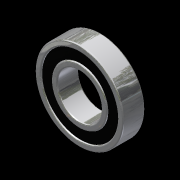
# Autodesk Inventor part: R8-2RS
Saved by Autodesk Inventor 2014 SP1 (Build 180222100, 222)
## iProperties
Created: 2014-04-23
Part Number: R8-2RS
Material: Generic
Document SubType Name: Modeling
Designer: Rauhul Varma
Density: 1 g/cm^3
Appearance: Default
Author: Rauhul Varma
Autodesk Inventor part; units mm, degrees
ref_plane "YZ Plane" through (0, 0, 0) normal (1, 0, 0) x (0, 1, 0)
ref_plane "XZ Plane" through (0, 0, 0) normal (0, 1, 0) x (-1, 0, 0)
ref_plane "XY Plane" through (0, 0, 0) normal (0, 0, 1) x (1, 0, 0)
sketch "Sketch1" plane through (0, 0, 0) normal (0, 0, 1) x (1, 0, 0)
  circle A0 centre (0, 0) radius 6
  circle A1 centre (0, 0) radius 12
  circle A2 centre (0, 0) radius 7.5875
  circle A3 centre (0, 0) radius 10.4125
  dimension "d0" = 12
  dimension "d1" = 24
  dimension "d2" = 15.175
  dimension "d3" = 1.5875
  constraints: 4 centre point, 4 coincident
  measures "d0" diameter of A0
  measures "d1" diameter of A1
  measures "d2" diameter of A2
  measures "d3" radial gap between concentric circles of A1 A3
extrude "Extrusion1" add sketch "Sketch1" along normal mid plane 6
extrude "Extrusion2" add sketch "Sketch1" along normal mid plane 5.2063 contours A3
fillet "Fillet1" radius 0.3969 8 edges at (-6, 0, 3) (-7.5875, 0, 3) (-10.4125, 0, 3) (-12, 0, 3) (-12, 0, -3) (-10.4125, 0, -3) (-7.5875, 0, -3) (-6, 0, -3)
equation "\"d2\" = d0 + 2 * d3"
body "Solid1"
